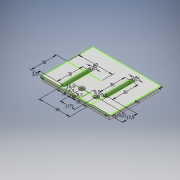
# Autodesk Inventor part: regla_digital2
Saved by Autodesk Inventor 2018 (Build 220112000, 112)
## iProperties
Created: 2019-02-11
Part Number: regla_digital2
Material: Generic
Document SubType Name: Modeling
Designer: zoticus
Density: 1 g/cm^3
Appearance: Default
Author: zoticus
Autodesk Inventor part; units mm, degrees
ref_plane "YZ Plane" through (0, 0, 0) normal (1, 0, 0) x (0, 1, 0)
ref_plane "XZ Plane" through (0, 0, 0) normal (0, 1, 0) x (-1, 0, 0)
ref_plane "XY Plane" through (0, 0, 0) normal (0, 0, 1) x (1, 0, 0)
sketch "Sketch1" plane through (0, 0, 0) normal (0, 0, 1) x (1, 0, 0)
  line L0 (-40, 30) -> (40, 30)
  line L1 (40, 30) -> (40, -30)
  line L2 (40, -30) -> (-40, -30)
  line L3 (-40, -30) -> (-40, 30)
  line L4 (-40, -30) -> (-40, 0)
  line L5 (-40, 0) -> (0, 0)
  line L6 (4.9275, -30) -> (4.9275, -19.5)
  line L7 (4.9275, -19.5) -> (13.4275, -19.5)
  line L8 (4.9275, -19.5) -> (-3.5725, -19.5)
  line L9 (0, -30) -> (-18, -30)
  line L10 (0, -30) -> (18, -30)
  line L11 (18, -30) -> (18, -12.5)
  line L12 (-18, -30) -> (-18, -26.5)
  line L13 (-18, -26.5) -> (-20.5, -26.5)
  line L14 (-20.5, -26.5) -> (-20.5, 3.5)
  line L15 (-20.5, 3.5) -> (-18, 3.5)
  line L16 (-18, 3.5) -> (-18, -26.5)
  line L17 (-18, -26.5) -> (-15.5, -26.5)
  line L18 (-15.5, -26.5) -> (-15.5, 3.5)
  line L19 (-15.5, 3.5) -> (-18, 3.5)
  line L20 (-18, 3.5) -> (-18, -26.5)
  line L21 (18, -12.5) -> (20.5, -12.5)
  line L22 (20.5, -12.5) -> (20.5, 17.5)
  line L23 (20.5, 17.5) -> (18, 17.5)
  line L24 (18, 17.5) -> (18, -12.5)
  line L25 (18, -12.5) -> (15.5, -12.5)
  line L26 (15.5, -12.5) -> (15.5, 17.5)
  line L27 (15.5, 17.5) -> (18, 17.5)
  line L28 (18, 17.5) -> (18, -12.5)
  line L29 (-3.5725, -19.5) -> (-10.0725, -19.5)
  line L30 (13.4275, -19.5) -> (19.9275, -19.5)
  point P0 (0, 0)
  dimension "d0" = 80
  dimension "d1" = 60
  dimension "d2" = 30
  dimension "d3" = 40
  dimension "d4" = 10.5
  dimension "d5" = 8.5
  dimension "d6" = 8.5
  dimension "d7" = 18
  dimension "d8" = 18
  dimension "d9" = 17.5
  dimension "d10" = 3.5
  dimension "d11" = 2.5
  dimension "d12" = 30
  dimension "d13" = 2.5
  dimension "d14" = 2.5
  dimension "d15" = 30
  dimension "d16" = 2.5
  dimension "d17" = 30
  dimension "d18" = 6.5
  dimension "d19" = 6.5
  dimension "d21" = 17
  dimension "d22" = 10.5
  dimension "d46" = 36
  constraints: 62 end point, 10 parallel, 8 horizontal, 8 perpendicular, 6 coincident, 3 point on line, 2 vertical, 1 midpoint
  measures "d0" distance of L1.end L2.end
  measures "d1" distance of L0.end L1.end
  measures "d2" distance of L2.end L4.end
  measures "d3" distance of L4.end L5.end
  measures "d4" distance of L6.start L6.end
  measures "d5" distance of L6.end L7.end
  measures "d6" distance of L6.end L8.end
  measures "d7" distance of L9.start L9.end
  measures "d8" distance of L10.start L10.end
  measures "d9" distance of L10.end L11.end
  measures "d10" distance of L9.end L12.end
  measures "d11" distance of L14.end L15.end
  measures "d12" distance of L13.end L14.end
  measures "d13" distance of L19.end L18.end
  measures "d14" distance of L23.end L22.end
  measures "d15" distance of L22.end L21.end
  measures "d16" distance of L26.end L27.end
  measures "d17" distance of L25.end L26.end
  measures "d18" distance of L29.start L29.end
  measures "d19" distance of L30.start L30.end
  measures "d21" distance of L7.end L8.end
  measures "d22" distance from line of L2 L7.end
  measures "d46" horizontal distance of L10.end point (-18, -26.5)
extrude "Extrusion1" add sketch "Sketch1" against normal blind 5 contours L0 L1 L2 L11 L30 L7 L6 L12 L17 L18 L19 L15 L14 L5 L3 | L5 L14 L13 L12 L2 L3 | L2 L6 L7 L30 L11
hole "Hole1" at (13.4275, -19.5, 0) at (-3.5725, -19.5, 0) direction (0, 0, -1) diameter 3 depth 10 counterbore diameter 6 counterbore depth 2.5
hole "Hole2" at (-18, -26.5, 0) at (-18, 3.5, 0) at (18, -12.5, 0) at (18, 17.5, 0) direction (0, 0, -1) diameter 5 depth 10 tip angle 118
sketch "Sketch2" plane through (13.4275, -19.5, -2.5) normal (0, 0, 1) x (1, 0, 0)
  point P0 (-13.4275, 19.5)
sketch "Sketch3" plane through (13.4275, -19.5, -2.5) normal (0, 0, 1) x (1, 0, 0)
  point P0 (-13.4275, 19.5)
body "Solid1"
